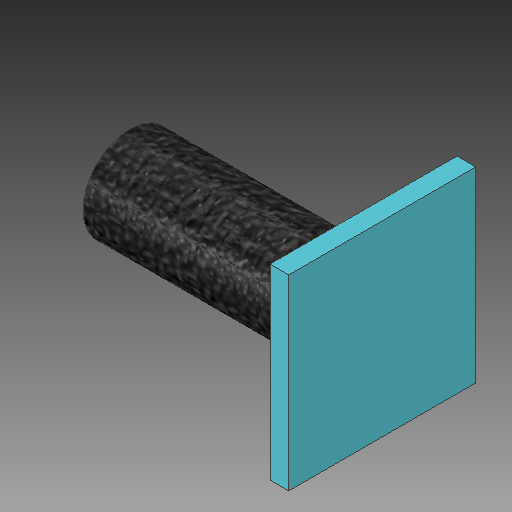
# Autodesk Inventor part: 激光传感器
Saved by Autodesk Inventor 2017 (Build 210142000, 142)
## iProperties
Part Number: 激光传感器
Material: 常规
Document SubType Name: Modeling
Designer: PANDA
Density: 1 g/cm^3
Appearance: 默认
Mass: 2.7635 g
Surface Area: 17.454 cm^2
Volume: 2.7635 cm^3
Author: PANDA
Autodesk Inventor part; units mm, degrees
ref_plane "YZ Plane" through (0, 0, 0) normal (1, 0, 0) x (0, 1, 0)
ref_plane "XZ Plane" through (0, 0, 0) normal (0, 1, 0) x (-1, 0, 0)
ref_plane "XY Plane" through (0, 0, 0) normal (0, 0, 1) x (1, 0, 0)
sketch "草图1" plane through (0, 0, 0) normal (1, 0, 0) x (0, 1, 0)
  circle A0 centre (0, 0) radius 5
  dimension "d0" = 10
  constraints: 1 centre point, 1 coincident
  measures "d0" diameter of A0
extrude "拉伸1" add sketch "草图1" along normal blind 15
sketch "草图2" plane through (15, 0, 0) normal (1, 0, 0) x (0, 0, -1)
  line L0 (10, 10) -> (-10, 10)
  line L1 (-10, 10) -> (-10, -10)
  line L2 (-10, -10) -> (10, -10)
  line L3 (10, -10) -> (10, 10)
  point P0 (0, 0)
  dimension "d3" = 20
  dimension "d4" = 20
  constraints: 8 end point, 2 parallel, 1 horizontal, 1 perpendicular
  measures "d3" distance of L2.end L1.end
  measures "d4" distance of L1.end L0.end
extrude "拉伸2" add sketch "草图2" along normal blind 2
sketch "草图3" plane through (0, 0, 0) normal (-1, 0, 0) x (0, 0, 1)
  circle A0 centre (0, 0) radius 5
  constraints: 1 centre point, 1 coincident
extrude "拉伸3" add sketch "草图3" along normal blind 10
